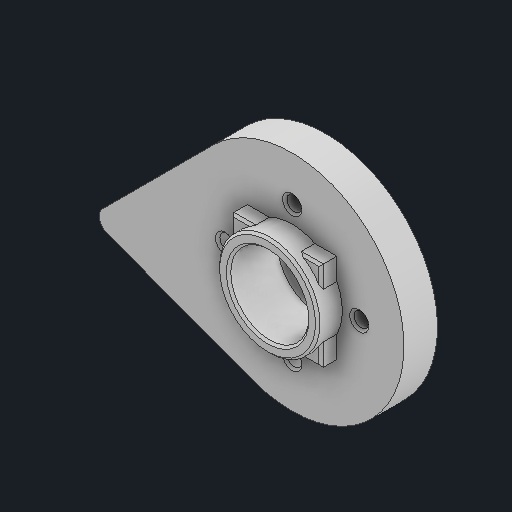
# Autodesk Inventor part: WeightBearingMount
Saved by Autodesk Inventor 2024.1 (Build 281209000, 209)
## iProperties
Created: 2023-10-16
Part Number: WeightBearingMount
Material: Generic
Document SubType Name: Modeling
Designer: Brandon
Density: 1 g/cm^3
Appearance: Default
Author: Brandon
Autodesk Inventor part; units mm, degrees
ref_plane "YZ Plane" through (0, 0, 0) normal (1, 0, 0) x (0, 1, 0)
ref_plane "XZ Plane" through (0, 0, 0) normal (0, 1, 0) x (-1, 0, 0)
ref_plane "XY Plane" through (0, 0, 0) normal (0, 0, 1) x (1, 0, 0)
ref_plane "Work Plane1" through (-0.0339, 0.0424, 0) normal (0, 0, 1) x (1, 0, 0)
sketch "Sketch1" plane through (-0.0339, 0.0424, 0) normal (0, 0, 1) x (1, 0, 0)
  circle A0 centre (-11, 0) radius 11 projected
  circle A1 centre (-11, 0) radius 11.0762
  arc A2 (-22.1037, -29.7451) -> (-33.4506, 22.4506) centre (-11, 0) ccw
  line L0 (1.7, 12.7) -> (-23.7, 12.7)
  line L1 (-23.7, 12.7) -> (-23.7, -12.7)
  line L2 (-23.7, -12.7) -> (1.7, -12.7)
  line L3 (1.7, -12.7) -> (1.7, 12.7)
  line L4 (1.7, 12.7) -> (-23.7, -12.7) construction
  line L5 (-23.7, 12.7) -> (1.7, -12.7) construction
  circle A3 centre (8.05, 0) radius 2.1
  circle A4 centre (-11, 19.05) radius 2.1
  circle A5 centre (-30.05, 0) radius 2.1
  circle A6 centre (-11, -19.05) radius 2.1
  circle A7 centre (-11, 0) radius 14.2512
  circle A8 centre (-11, 0) radius 4.35
  line L6 (-33.4506, 22.4506) -> (-64.8815, -8.9803)
  arc A9 (-64.8815, -8.9803) -> (-63.7468, -14.1998) centre (-62.6365, -11.2253) ccw
  line L7 (-22.1037, -29.7451) -> (-63.7468, -14.1998)
  line L8 (-46.921, 8.9803) -> (-64.8815, -8.9803)
  point P0 (0.0339, -0.0424)
  point P1 (-23.7, 6.4658)
  point P2 (-17.4658, 12.7)
  point P3 (-17.4658, -12.7)
  point P4 (-23.7, -6.4658)
  point P5 (1.7, -6.4658)
  point P6 (-4.5342, -12.7)
  point P7 (-4.5342, 12.7)
  point P8 (1.7, 6.4658)
  point P9 (-42.4309, 4.4901)
  dimension "d0" = 0.0762
  dimension "d1" = 63.5
  dimension "d2" = 25.4
  dimension "d3" = 25.4
  dimension "d4" = 4.2
  dimension "d5" = 19.05
  dimension "d8" = 360
  dimension "d10" = 3.175
  dimension "d15" = 8.7
  dimension "d23" = 6.35
  constraints: 18 end point, 9 centre point, 5 point on circle, 3 coincident, 3 tangent, 2 midpoint, 2 parallel, 1 horizontal, 1 horizontal alignment, 1 perpendicular, 1 point on line, 13 other
  measures "d1" diameter of A2
  measures "d2" distance of L2.end L1.end
  measures "d3" distance of L1.end L0.end
  measures "d4" diameter of A3
  measures "d5" distance of A1.centre A3.centre
  measures "d10" radial gap between concentric circles of A1 A7
  measures "d15" diameter of A8
  measures "d23" diameter of A9
extrude "Extrusion1" add sketch "Sketch1" along normal blind 16.505 contours A7 L3 L2 L1 L0 | L0 A7 | A7 L3 | L1 A7 | A7 L2
extrude "Extrusion2" add sketch "Sketch1" along normal blind 9.525 contours L7 A9 L6 A2 | L3 A7 L0 | A7 L3 L2 L1 L0 | L0 A7 | A7 L3 | A7 L1 L0 | L3 L2 A7 | L1 A7 | A7 L2 | A7 L2 L1
extrude "Extrusion3" add sketch "Sketch1" along normal blind 2.505 contours A0 | A1
extrude "Extrusion4" add sketch "Sketch1" along normal blind 13.97 contours L3 A7 L0 | A7 L1 L0 | L3 L2 A7 | A7 L2 L1
chamfer "Chamfer1" distance 0.635 angle 45 14 edges at (-22.1101, 0.0424, 16.505) (5.9161, 0.0424, 9.525) (-13.1339, 19.0924, 9.525) (-13.1339, -19.0076, 9.525) (-32.1839, 0.0424, 9.525) (1.6661, 9.6253, 13.97) (-1.451, 12.7424, 13.97) (-20.6168, 12.7424, 13.97) (-23.7339, 9.6253, 13.97) (1.6661, -9.5405, 13.97) (-1.451, -12.6576, 13.97) (-23.7339, -9.5405, 13.97) (-20.6168, -12.6576, 13.97) (-25.2851, 0.0424, 16.505)
body "Solid1"
